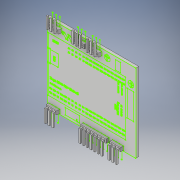
# Autodesk Inventor part: board_v2
Saved by Autodesk Inventor 2019 (Build 230136000, 136)
## iProperties
Created: 2020-03-31
Part Number: board_v2
Material: Generic
Document SubType Name: Modeling
Designer: Pulag
Density: 1 g/cm^3
Appearance: Default
Autodesk Inventor part; units mm, degrees
note: some values were not read from the file. Chosen so that the rebuilt part matches the saved one: hole positions of "Sketch Driven Pattern2".
ref_plane "YZ Plane" through (0, 0, 0) normal (1, 0, 0) x (0, 1, 0)
ref_plane "XZ Plane" through (0, 0, 0) normal (0, 1, 0) x (-1, 0, 0)
ref_plane "XY Plane" through (0, 0, 0) normal (0, 0, 1) x (1, 0, 0)
sketch "Sketch1" plane through (0, 0, 0) normal (0, 0, 1) x (1, 0, 0)
  point P0 (0, 0)
sketch3d "3D 20"
sketch3d "3D 21"
sketch3d "3D 51"
sketch "Sketch2" plane through (0, 0, 0) normal (0, 0, 1) x (1, 0, 0)
  line L0 (0, 54.6) -> (61.9, 54.6)
  line L1 (61.9, 54.6) -> (61.9, 0)
  line L2 (61.9, 0) -> (0, 0)
  line L3 (0, 0) -> (0, 54.6)
  constraints: 8 end point, 2 parallel, 1 horizontal, 1 perpendicular
extrude "PCB" add sketch "Sketch2" against normal blind 2
sketch "Sketch3" plane through (0, 0, 0) normal (0, 0, 1) x (1, 0, 0)
  line L0 (38.1, 50.165) -> (38.1, 52.705) projected
  line L1 (38.1, 52.705) -> (35.56, 52.705) projected
  line L2 (35.56, 50.165) -> (38.1, 50.165) projected
  line L3 (35.56, 50.165) -> (35.56, 52.705) projected
  line L4 (35.56, 52.705) -> (33.02, 52.705) projected
  line L5 (33.02, 50.165) -> (35.56, 50.165) projected
  line L6 (33.02, 50.165) -> (33.02, 52.705) projected
  line L7 (33.02, 52.705) -> (30.48, 52.705) projected
  line L8 (30.48, 50.165) -> (33.02, 50.165) projected
  line L9 (30.48, 52.705) -> (30.48, 50.165) projected
  line L10 (27.94, 52.705) -> (25.4, 52.705) projected
  line L11 (27.94, 50.165) -> (27.94, 52.705) projected
  line L12 (25.4, 50.165) -> (27.94, 50.165) projected
  line L13 (25.4, 50.165) -> (25.4, 52.705) projected
  line L14 (25.4, 52.705) -> (22.86, 52.705) projected
  line L15 (22.86, 50.165) -> (25.4, 50.165) projected
  line L16 (0, 54.6) -> (61.9, 54.6) projected
  line L17 (0, 0) -> (0, 54.6) projected
  line L18 (61.9, 0) -> (0, 0) projected
  line L19 (61.9, 54.6) -> (61.9, 0) projected
  line L20 (22.86, 50.165) -> (22.86, 52.705) projected
  line L21 (22.86, 52.705) -> (20.32, 52.705) projected
  line L22 (20.32, 50.165) -> (22.86, 50.165) projected
  line L23 (20.32, 52.705) -> (20.32, 50.165) projected
  line L24 (10.16, 52.705) -> (7.62, 52.705) projected
  line L25 (10.16, 50.165) -> (10.16, 52.705) projected
  line L26 (7.62, 50.165) -> (10.16, 50.165) projected
  line L27 (7.62, 50.165) -> (7.62, 52.705) projected
  line L28 (7.62, 52.705) -> (5.08, 52.705) projected
  line L29 (5.08, 50.165) -> (7.62, 50.165) projected
  line L30 (5.08, 50.165) -> (5.08, 52.705) projected
  line L31 (5.08, 52.705) -> (2.54, 52.705) projected
  line L32 (2.54, 50.165) -> (5.08, 50.165) projected
  line L33 (2.54, 52.705) -> (2.54, 50.165) projected
  line L34 (8.89, 0.635) -> (8.89, 3.175) projected
  line L35 (8.89, 3.175) -> (6.35, 3.175) projected
  line L36 (6.35, 0.635) -> (8.89, 0.635) projected
  line L37 (6.35, 3.175) -> (6.35, 0.635) projected
  line L38 (6.35, 3.175) -> (3.81, 3.175) projected
  line L39 (3.81, 0.635) -> (6.35, 0.635) projected
  line L40 (3.81, 3.175) -> (3.81, 0.635) projected
  line L41 (3.81, 3.175) -> (1.27, 3.175) projected
  line L42 (1.27, 0.635) -> (3.81, 0.635) projected
  line L43 (1.27, 3.175) -> (1.27, 0.635) projected
  line L44 (25.4, 3.175) -> (25.4, 0.635) projected
  line L45 (27.94, 3.175) -> (25.4, 3.175) projected
  line L46 (25.4, 0.635) -> (27.94, 0.635) projected
  line L47 (27.94, 3.175) -> (27.94, 0.635) projected
  line L48 (30.48, 3.175) -> (27.94, 3.175) projected
  line L49 (27.94, 0.635) -> (30.48, 0.635) projected
  line L50 (30.48, 3.175) -> (30.48, 0.635) projected
  line L51 (33.02, 3.175) -> (30.48, 3.175) projected
  line L52 (30.48, 0.635) -> (33.02, 0.635) projected
  line L53 (33.02, 3.175) -> (33.02, 0.635) projected
  line L54 (35.56, 3.175) -> (33.02, 3.175) projected
  line L55 (33.02, 0.635) -> (35.56, 0.635) projected
  line L56 (35.56, 3.175) -> (35.56, 0.635) projected
  line L57 (38.1, 3.175) -> (35.56, 3.175) projected
  line L58 (35.56, 0.635) -> (38.1, 0.635) projected
  line L59 (38.1, 3.175) -> (38.1, 0.635) projected
  line L60 (40.64, 3.175) -> (38.1, 3.175) projected
  line L61 (40.64, 3.175) -> (40.64, 0.635) projected
  line L62 (38.1, 0.635) -> (40.64, 0.635) projected
  line L63 (43.18, 3.175) -> (40.64, 3.175) projected
  line L64 (43.18, 0.635) -> (43.18, 3.175) projected
  line L65 (40.64, 0.635) -> (43.18, 0.635) projected
  line L66 (45.72, 3.175) -> (45.72, 0.635) projected
  line L67 (48.26, 3.175) -> (45.72, 3.175) projected
  line L68 (45.72, 0.635) -> (48.26, 0.635) projected
  line L69 (48.26, 3.175) -> (48.26, 0.635) projected
  line L70 (50.8, 3.175) -> (48.26, 3.175) projected
  line L71 (48.26, 0.635) -> (50.8, 0.635) projected
  line L72 (50.8, 3.175) -> (50.8, 0.635) projected
  line L73 (53.34, 3.175) -> (50.8, 3.175) projected
  line L74 (50.8, 0.635) -> (53.34, 0.635) projected
  line L75 (53.34, 0.635) -> (53.34, 3.175) projected
extrude "PIN_1" add sketch "Sketch3" along normal blind 2 contours L2 L3 L1 L0
sketch "Sketch4" plane through (0, 0, 2) normal (0, 0, 1) x (1, 0, 0)
  line L0 (38.1, 52.705) -> (38.1, 50.165) projected
  line L1 (35.56, 50.165) -> (35.56, 52.705) projected
  line L2 (38.1, 52.705) -> (35.56, 50.165)
  line L3 (36.33, 51.935) -> (37.33, 51.935)
  line L4 (37.33, 51.935) -> (37.33, 50.935)
  line L5 (37.33, 50.935) -> (36.33, 50.935)
  line L6 (36.33, 50.935) -> (36.33, 51.935)
  line L7 (36.33, 51.935) -> (37.33, 50.935) construction
  line L8 (37.33, 51.935) -> (36.33, 50.935) construction
  point P0 (0, 0)
  point P1 (36.83, 51.435)
  dimension "d4" = 1
  dimension "d5" = 1
  constraints: 14 end point, 3 midpoint, 2 parallel, 1 horizontal, 1 perpendicular
  measures "d4" distance of L4.end L5.end
  measures "d5" distance of L3.end L4.end
extrude "PIN_2" add sketch "Sketch4" along normal blind 2
sketch "Sketch5" plane through (36.33, 51.935, 2) normal (0, 1, 0) x (1, 0, 0)
  line L0 (1, 0) -> (1, -2) projected
  line L1 (1, -1) -> (0, -1)
  line L2 (0, 0) -> (0, -2) projected
  line L3 (0, -1) -> (1, -1)
  line L4 (1, -1) -> (1, -2)
  line L5 (1, -2) -> (0, -2)
  line L6 (0, -2) -> (0, -1)
  line L7 (0, -1) -> (1, -2) construction
  line L8 (1, -1) -> (0, -2) construction
  point P0 (-36.33, 2)
  point P1 (0.5, -1.5)
  dimension "d8" = 1
  dimension "d9" = 1
  constraints: 14 end point, 4 midpoint, 2 parallel, 1 horizontal, 1 perpendicular
  measures "d8" distance of L0.end L5.end
  measures "d9" distance of L3.end L0.end
extrude "PIN_3" add sketch "Sketch5" along normal blind 7
sketch "Sketch7" plane through (0, 0, 0) normal (0, 0, 1) x (1, 0, 0)
  line L0 (33.02, 50.165) -> (35.56, 50.165) projected
  line L1 (38.1, 50.165) -> (35.56, 50.165) projected
  line L2 (35.56, 50.165) -> (35.56, 52.705) projected
  line L3 (35.56, 52.705) -> (38.1, 52.705) projected
  line L4 (38.1, 52.705) -> (38.1, 50.165) projected
  line L5 (0, 54.6) -> (61.9, 54.6) projected
  line L6 (0, 0) -> (0, 54.6) projected
  line L7 (61.9, 0) -> (0, 0) projected
  line L8 (61.9, 54.6) -> (61.9, 0) projected
  line L9 (30.48, 50.165) -> (33.02, 50.165) projected
  line L10 (25.4, 50.165) -> (27.94, 50.165) projected
  line L11 (22.86, 50.165) -> (25.4, 50.165) projected
  line L12 (20.32, 50.165) -> (22.86, 50.165) projected
  line L13 (7.62, 50.165) -> (10.16, 50.165) projected
  line L14 (5.08, 50.165) -> (7.62, 50.165) projected
  line L15 (2.54, 50.165) -> (5.08, 50.165) projected
  point P0 (3.81, 50.165)
  point P1 (6.35, 50.165)
  point P2 (8.89, 50.165)
  point P3 (21.59, 50.165)
  point P4 (24.13, 50.165)
  point P5 (26.67, 50.165)
  point P6 (31.75, 50.165)
  point P7 (34.29, 50.165)
  constraints: 8 midpoint
pattern_sketch "Sketch Driven Pattern1" of "PIN_1", "PIN_2", "PIN_3" from (36.83, 50.165, 0) copies at (3.81, 50.165, 0) at (6.35, 50.165, 0) at (8.89, 50.165, 0) at (21.59, 50.165, 0) at (24.13, 50.165, 0) at (26.67, 50.165, 0) at (31.75, 50.165, 0) at (34.29, 50.165, 0)
sketch "Sketch8" plane through (0, 0, 0) normal (0, 0, 1) x (1, 0, 0)
  line L0 (53.34, 3.175) -> (50.8, 3.175) projected
  line L1 (50.8, 3.175) -> (48.26, 3.175) projected
  line L2 (48.26, 3.175) -> (45.72, 3.175) projected
  line L3 (43.18, 3.175) -> (40.64, 3.175) projected
  line L4 (40.64, 3.175) -> (38.1, 3.175) projected
  line L5 (38.1, 3.175) -> (35.56, 3.175) projected
  line L6 (35.56, 3.175) -> (33.02, 3.175) projected
  line L7 (33.02, 3.175) -> (30.48, 3.175) projected
  line L8 (30.48, 3.175) -> (27.94, 3.175) projected
  line L9 (27.94, 3.175) -> (25.4, 3.175) projected
  line L10 (8.89, 3.175) -> (6.35, 3.175) projected
  line L11 (6.35, 3.175) -> (3.81, 3.175) projected
  line L12 (3.81, 3.175) -> (1.27, 3.175) projected
  point P0 (0, 0)
  point P1 (2.54, 3.175)
  point P2 (5.08, 3.175)
  point P3 (7.62, 3.175)
  point P4 (26.67, 3.175)
  point P5 (29.21, 3.175)
  point P6 (31.75, 3.175)
  point P7 (34.29, 3.175)
  point P8 (36.83, 3.175)
  point P9 (39.37, 3.175)
  point P10 (41.91, 3.175)
  point P11 (46.99, 3.175)
  point P12 (49.53, 3.175)
  point P13 (52.07, 3.175)
  constraints: 13 midpoint
sketch "Sketch9" plane through (0, 0, 0) normal (0, 0, 1) x (1, 0, 0)
  line L0 (1.3081, 0.635) -> (3.8481, 0.635)
  line L1 (3.8481, 0.635) -> (3.8481, 3.175)
  line L2 (3.8481, 3.175) -> (1.3081, 3.175)
  line L3 (1.3081, 3.175) -> (1.3081, 0.635)
  point P0 (0, 0)
  constraints: 8 end point, 2 parallel, 1 horizontal, 1 perpendicular
extrude "Extrusion5" add sketch "Sketch9" along normal blind 2
sketch "Sketch10" plane through (0, 0, 2) normal (0, 0, 1) x (1, 0, 0)
  line L0 (3.8481, 3.175) -> (3.8481, 0.635) projected
  line L1 (1.3081, 3.175) -> (1.3081, 0.635) projected
  line L2 (2.0781, 2.405) -> (3.0781, 2.405)
  line L3 (3.0781, 2.405) -> (3.0781, 1.405)
  line L4 (3.0781, 1.405) -> (2.0781, 1.405)
  line L5 (2.0781, 1.405) -> (2.0781, 2.405)
  line L6 (2.0781, 2.405) -> (3.0781, 1.405) construction
  line L7 (3.0781, 2.405) -> (2.0781, 1.405) construction
  point P0 (0, 0)
  point P1 (2.5781, 1.905)
  dimension "d14" = 1
  dimension "d15" = 1
  constraints: 12 end point, 2 midpoint, 2 parallel, 1 horizontal, 1 perpendicular
  measures "d14" distance of L3.end L4.end
  measures "d15" distance of L2.end L3.end
extrude "Extrusion6" add sketch "Sketch10" along normal blind 2
sketch "Sketch11" plane through (2.0781, 1.405, 2) normal (0, -1, 0) x (1, 0, 0)
  line L0 (1, 2) -> (0, 2) projected
  line L1 (1, 2) -> (0, 2)
  line L2 (0, 2) -> (0, 1)
  line L3 (0, 1) -> (1, 1)
  line L4 (1, 1) -> (1, 2)
  point P0 (-2.0781, -2)
  dimension "d18" = 1
  dimension "d19" = 1
  constraints: 8 end point, 2 parallel, 1 horizontal, 1 perpendicular
  measures "d18" distance of L3.end L2.end
  measures "d19" distance of L2.end L1.end
extrude "Extrusion7" add sketch "Sketch11" along normal blind 8
pattern_sketch "Sketch Driven Pattern2" of "Extrusion5", "Extrusion6", "Extrusion7" from (2.5781, 3.175, 0) copies at (2.54, 3.175, 0) at (5.08, 3.175, 0) at (7.62, 3.175, 0) at (26.67, 3.175, 0) at (29.21, 3.175, 0) at (31.75, 3.175, 0) at (34.29, 3.175, 0) at (36.83, 3.175, 0) at (39.37, 3.175, 0) at (41.91, 3.175, 0) at (46.99, 3.175, 0) at (49.53, 3.175, 0) at (52.07, 3.175, 0)
body "Solid1"
